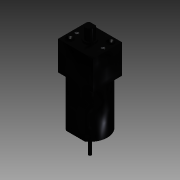
# Autodesk Inventor part: Motor XDRIVE GM12F
Saved by Autodesk Inventor 2014 SP1 (Build 180222100, 222)
## iProperties
Created: 2013-08-08
Part Number: Motor XDRIVE GM12F
Material: Allgemein
Document SubType Name: Modeling
Designer: vogel
Density: 1 g/cm^3
Appearance: Schwarz
Author: vogel
Autodesk Inventor part; units mm, degrees
ref_plane "YZ Plane" through (0, 0, 0) normal (1, 0, 0) x (0, 1, 0)
ref_plane "XZ Plane" through (0, 0, 0) normal (0, 1, 0) x (-1, 0, 0)
ref_plane "XY Plane" through (0, 0, 0) normal (0, 0, 1) x (1, 0, 0)
sketch "Skizze1" plane through (0, 0, 0) normal (0, 0, 1) x (1, 0, 0)
  line L0 (-8.4, 0) -> (8.4, 0) projected
  line L1 (0, -7) -> (0, 7) projected
  line L2 (-6, 5) -> (6, 5)
  line L3 (6, 5) -> (6, -5)
  line L4 (6, -5) -> (-6, -5)
  line L5 (-6, -5) -> (-6, 5)
  point P0 (0, 0)
  dimension "d0" = 10
  dimension "d1" = 12
  constraints: 8 end point, 2 parallel, 1 horizontal, 1 perpendicular, 2 other
  measures "d0" distance of L4.end L2.start
  measures "d1" distance of L2.start L2.end
extrude "Extrusion1" add sketch "Skizze1" along normal blind 26
sketch "Skizze2" plane through (0, 0, 26) normal (0, 0, 1) x (1, 0, 0)
  circle A0 centre (0, 0) radius 2
  dimension "d4" = 4
  constraints: 1 centre point, 1 coincident
  measures "d4" diameter of A0
extrude "Extrusion2" add sketch "Skizze2" along normal blind 0.65
sketch "Skizze3" plane through (0, 0, 26) normal (0, 0, 1) x (1, 0, 0)
  circle A0 centre (0, 0) radius 2 projected
  circle A1 centre (0, 0) radius 1.5
  dimension "d7" = 3
  constraints: 1 centre point, 1 coincident
  measures "d7" diameter of A1
extrude "Extrusion3" add sketch "Skizze3" along normal blind 4.5 contours A1
sketch "Skizze4" plane through (0, 0, 26) normal (0, 0, 1) x (1, 0, 0)
  line L0 (-8.4, 0) -> (8.4, 0) projected
  line L1 (0, -7) -> (0, 7) projected
  line L2 (-4, 3) -> (4, 3)
  line L3 (4, 3) -> (4, -3)
  line L4 (4, -3) -> (-4, -3)
  line L5 (-4, -3) -> (-4, 3)
  dimension "d10" = 6
  dimension "d11" = 8
  constraints: 8 end point, 2 coincident, 2 parallel, 1 horizontal, 1 perpendicular, 2 other
  measures "d10" distance of L4.end L2.start
  measures "d11" distance of L3.end L4.end
hole "Bohrung1" at (-4, -3, 26) at (4, 3, 26) at (-4, -3, 26) at (4, 3, 26) direction (0, 0, -1) diameter 1.4 depth 8 tip angle 118 countersink diameter 2.5 countersink angle 90
sketch "Skizze5" plane through (0, 0, 26) normal (0, 0, 1) x (1, 0, 0)
  line L0 (-8.4, 0) -> (8.4, 0) projected
  line L1 (0, -7) -> (0, 7) projected
  point P0 (-4.5, 0)
  point P1 (4.5, 0)
  dimension "d19" = 9
  constraints: 2 point on line, 1 symmetric about line
  measures "d19" distance of point (4.5, 0) point (-4.5, 0)
hole "Bohrung2" at (-4.5, 0, 26) at (4.5, 0, 26) direction (0, 0, -1) diameter 1.221 depth 8 tip angle 118 thread size "M1.6x0.35" class "6H" standard "ISO Metric profile"
sketch "Skizze6" plane through (0, 0, 0) normal (0, 0, -1) x (-1, 0, 0)
  circle A0 centre (0, 0) radius 0.5
  dimension "d27" = 1
  constraints: 1 centre point, 1 coincident
  measures "d27" diameter of A0
extrude "Extrusion4" add sketch "Skizze6" along normal blind 8
sketch "Skizze8" plane through (0, 0, 0) normal (0, 0, -1) x (-1, 0, 0)
  circle A0 centre (0, 0) radius 0.5 projected
  line L0 (6, 5) -> (-6, 5) projected
  line L1 (-6, 5) -> (-6, -5) projected
  line L2 (-6, -5) -> (6, -5) projected
  line L3 (6, -5) -> (6, 5) projected
  arc A1 (-3.2253, 5) -> (-3.2253, -5) centre (0, 0) ccw
  arc A2 (3.2253, -5) -> (3.2253, 5) centre (0, 0) ccw
  dimension "d38" = 5.95
  dimension "d39" = 5.95
  constraints: 4 point on circle, 4 point on line, 2 centre point, 1 coincident
  measures "d38" radius of A1
  measures "d39" radius of A2
extrude "Extrusion6" cut sketch "Skizze8" against normal blind 16 contours L3 L2 A2 L0 | A1 L2 L1 L0
sketch "Skizze9" plane through (0, 0, 30.5) normal (0, 0, 1) x (1, 0, 0)
  circle A0 centre (0, 0) radius 1.5 projected
  line L0 (-1.118, 1) -> (1.118, 1)
  dimension "d42" = 1
  constraints: 2 end point, 2 point on circle, 1 horizontal
  measures "d42" distance from line of L0 A0.centre
extrude "Extrusion7" cut sketch "Skizze9" against normal up to surface (3.85 mm away) contours L0 A0 picked at (-0.0599, 1.1631)
